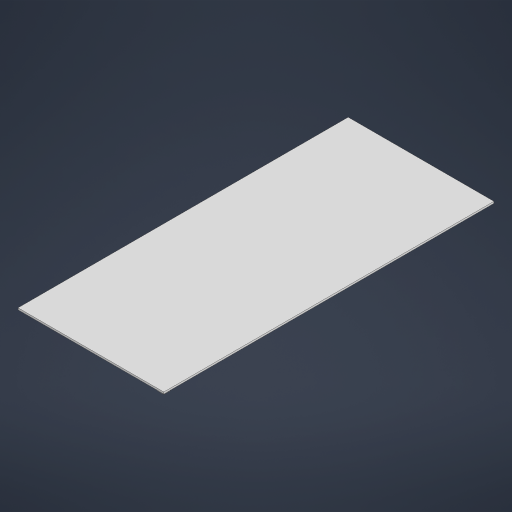
# Autodesk Inventor part: Tabla
Saved by Autodesk Inventor 2024 (Build 280153000, 153)
## iProperties
Created: 2023-04-23
Part Number: Tabla
Material: Genérico
Document SubType Name: Modeling
Designer: javie
Density: 1 g/cm^3
Appearance: Valor por defecto
Author: javie
Autodesk Inventor part; units mm, degrees
ref_plane "YZ Plane" through (0, 0, 0) normal (1, 0, 0) x (0, 1, 0)
ref_plane "XZ Plane" through (0, 0, 0) normal (0, 1, 0) x (-1, 0, 0)
ref_plane "XY Plane" through (0, 0, 0) normal (0, 0, 1) x (1, 0, 0)
sketch "Boceto1" plane through (0, 0, 0) normal (0, 1, 0) x (-1, 0, 0)
  line L0 (0, 0) -> (-830, 0)
  line L1 (-830, 0) -> (-830, -1880)
  line L2 (-830, -1880) -> (0, -1880)
  line L3 (0, -1880) -> (0, 0)
  dimension "d0" = 830
  dimension "d1" = 1880
  constraints: 8 end point, 2 parallel, 1 horizontal, 1 perpendicular
  measures "d0" distance of L2.end L1.end
  measures "d1" distance of L1.end L0.end
extrude "Extrusión1" add sketch "Boceto1" along normal blind 10
sketch "Boceto2" plane through (0, 0, 0) normal (0, -1, 0) x (1, 0, 0)
  line L0 (828.5, -1.5) -> (791.5, -1.5)
  line L1 (791.5, -1.5) -> (791.5, -38.5)
  line L2 (791.5, -38.5) -> (828.5, -38.5)
  line L3 (828.5, -38.5) -> (828.5, -1.5)
  line L4 (0, 0) -> (830, 0) projected
  line L5 (830, 0) -> (830, -1880) projected
  dimension "d4" = 37
  dimension "d5" = 37
  dimension "d6" = 1.5
  dimension "d7" = 1.5
  constraints: 8 end point, 2 parallel, 1 horizontal, 1 perpendicular
  measures "d4" distance of L2.end L1.end
  measures "d5" distance of L1.end L0.end
  measures "d6" distance between parallel lines of L4 L0
  measures "d7" distance between parallel lines of L5 L3
extrude "Extrusión2" add sketch "Boceto2" along normal blind 4
